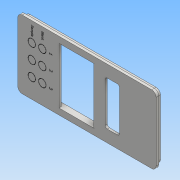
# Autodesk Inventor part: Box2_top
Saved by Autodesk Inventor 2016 (Build 200138000, 138)
## iProperties
Created: 2015-09-13
Part Number: Box2_top
Material: PPS Plastic
Document SubType Name: Modeling
Designer: Openlab
Density: 1.637 g/cm^3
Appearance: White
Mass: 58.6735 g
Surface Area: 261.578 cm^2
Volume: 35.8421 cm^3
Author: Openlab
Autodesk Inventor part; units mm, degrees
(part 1 of 2)
ref_plane "YZ Plane" through (0, 0, 0) normal (1, 0, 0) x (0, 1, 0)
ref_plane "XZ Plane" through (0, 0, 0) normal (0, 1, 0) x (-1, 0, 0)
ref_plane "XY Plane" through (0, 0, 0) normal (0, 0, 1) x (1, 0, 0)
sketch "Sketch1" plane through (0, 0, 0) normal (0, 1, 0) x (-1, 0, 0)
  line L0 (-70, 35) -> (70, 35)
  line L1 (75, 30) -> (75, -30)
  line L2 (70, -35) -> (-70, -35)
  line L3 (-75, -30) -> (-75, 30)
  line L4 (-75, 35) -> (75, -35) construction
  line L5 (75, 35) -> (-75, -35) construction
  arc A0 (75, 30) -> (70, 35) centre (70, 30) ccw
  arc A1 (70, -35) -> (75, -30) centre (70, -30) ccw
  arc A2 (-70, 35) -> (-75, 30) centre (-70, 30) ccw
  arc A3 (-75, -30) -> (-70, -35) centre (-70, -30) ccw
  line L6 (-72, 37) -> (72, 37)
  line L7 (77, 32) -> (77, -32)
  line L8 (72, -37) -> (-72, -37)
  line L9 (-77, -32) -> (-77, 32)
  line L10 (-77, 37) -> (77, -37) construction
  line L11 (77, 37) -> (-77, -37) construction
  arc A4 (77, 32) -> (72, 37) centre (72, 32) ccw
  arc A5 (72, -37) -> (77, -32) centre (72, -32) ccw
  arc A6 (-77, -32) -> (-72, -37) centre (-72, -32) ccw
  arc A7 (-72, 37) -> (-77, 32) centre (-72, 32) ccw
  line L12 (74, 39) -> (-74, 39)
  line L13 (-79, 34) -> (-79, -34)
  line L14 (-74, -39) -> (74, -39)
  line L15 (79, -34) -> (79, 34)
  line L16 (79, 39) -> (-79, -39) construction
  line L17 (-79, 39) -> (79, -39) construction
  arc A8 (79, 34) -> (74, 39) centre (74, 34) ccw
  arc A9 (-74, 39) -> (-79, 34) centre (-74, 34) ccw
  arc A10 (-79, -34) -> (-74, -39) centre (-74, -34) ccw
  arc A11 (74, -39) -> (79, -34) centre (74, -34) ccw
  line L18 (-22.75, 23.25) -> (-35.25, 23.25) construction
  line L19 (-35.25, 23.25) -> (-35.25, 19) construction
  line L20 (-35.25, 10.75) -> (-22.75, 10.75) construction
  line L21 (-22.75, 10.75) -> (-22.75, 15) construction
  line L22 (56.9183, 17) -> (21.35, 17) construction
  line L23 (40.8, -24) -> (40.8, -20.1) construction
  line L24 (-55.8, 24) -> (-55.8, 12) construction
  line L25 (-20.25, 15.5) -> (-22.25, 15.5) construction
  line L26 (-22.25, 18.5) -> (-20.25, 18.5) construction
  line L27 (-35.75, 15.5) -> (-37.75, 15.5) construction
  line L28 (-37.75, 18.5) -> (-35.75, 18.5) construction
  line L29 (-40.55, 18.5) -> (-53.5, 18.5) construction
  line L30 (-40.55, 15.5) -> (-53.5, 15.5) construction
  line L31 (-60, 8.5) -> (45, 8.5) construction
  line L32 (38.5, 20.5) -> (37, 20.5) construction
  line L33 (37, 13.5) -> (38.5, 13.5) construction
  line L34 (-60, 5) -> (-60, -25) construction
  line L35 (21.35, -8.5) -> (45, -8.5) construction
  line L36 (-29, 20.0147) -> (-29, -25.5) construction
  line L37 (31.2062, 0) -> (-4.2501, 0) construction
  line L38 (-35.25, 6.25) -> (-35.25, 2) construction
  line L39 (-22.75, 6.25) -> (-35.25, 6.25) construction
  line L40 (-22.75, -6.25) -> (-22.75, -2) construction
  line L41 (-35.25, -6.25) -> (-22.75, -6.25) construction
  line L42 (-22.25, 1.5) -> (-20.25, 1.5) construction
  line L43 (-20.25, -1.5) -> (-22.25, -1.5) construction
  line L44 (38.5, 3.5) -> (37, 3.5) construction
  line L45 (37, -3.5) -> (38.5, -3.5) construction
  line L46 (-22.75, -10.75) -> (-35.25, -10.75) construction
  line L47 (-22.75, -23.25) -> (-22.75, -19) construction
  line L48 (-35.25, -23.25) -> (-22.75, -23.25) construction
  line L49 (56.3008, -17) -> (21.35, -17) construction
  line L50 (38.5, -13.5) -> (37, -13.5) construction
  line L51 (37, -20.5) -> (38.5, -20.5) construction
  line L52 (-20.25, -18.5) -> (-22.25, -18.5) construction
  line L53 (44.5, 5.5) -> (43.5, 5.5) construction
  line L54 (41.3, 11.5) -> (43.5, 11.5) construction
  line L55 (-37.75, -15.5) -> (-35.75, -15.5) construction
  line L56 (-35.75, -18.5) -> (-37.75, -18.5) construction
  line L57 (-40.55, -18.5) -> (-53.5, -18.5) construction
  line L58 (-37.75, 1.5) -> (-35.75, 1.5) construction
  line L59 (-35.75, -1.5) -> (-37.75, -1.5) construction
  line L60 (-40.55, -1.5) -> (-53.5, -1.5) construction
  line L61 (-58.5, 5.5) -> (-59.5, 5.5) construction
  line L62 (-59.5, 11.5) -> (-58.5, 11.5) construction
  line L63 (38.5, 5.5) -> (37, 5.5) construction
  line L64 (37, 5.5) -> (37, 11.5) construction
  line L65 (37, 11.5) -> (38.5, 11.5) construction
  line L66 (-53.5, 5.5) -> (-52.5, 5.5) construction
  line L67 (-52.5, 5.5) -> (-52.5, 11.5) construction
  line L68 (-52.5, 11.5) -> (-53.5, 11.5) construction
  line L69 (-54, 24) -> (-54, 19) construction
  line L70 (-54, 5) -> (-54, 2) construction
  arc A12 (-12.95, 13.5) -> (-12.95, 3.5) centre (-12.95, 8.5) ccw construction
  arc A13 (31, 3.5) -> (31, 13.5) centre (31, 8.5) ccw construction
  arc A14 (-12.95, -3.5) -> (-12.95, -13.5) centre (-12.95, -8.5) ccw construction
  arc A15 (31, -13.5) -> (31, -3.5) centre (31, -8.5) ccw construction
  line L71 (-12.95, 13.5) -> (31, 13.5) construction
  line L72 (-12.95, 3.5) -> (31, 3.5) construction
  line L73 (-12.95, -3.5) -> (31, -3.5) construction
  line L74 (-12.95, -13.5) -> (31, -13.5) construction
  arc A16 (-45.05, -13.5) -> (-45.05, -3.5) centre (-45.05, -8.5) ccw construction
  line L75 (43.5, -24) -> (43.5, -19.6) construction
  line L76 (-58.5, 24) -> (-58.5, 11.5) construction
  arc A17 (-46, -3.5) -> (-46, -13.5) centre (-46, -8.5) ccw construction
  arc A18 (-46, 13.5) -> (-46, 3.5) centre (-46, 8.5) ccw construction
  line L77 (-45.05, -13.5) -> (-46, -13.5) construction
  line L78 (-46, -3.5) -> (-45.05, -3.5) construction
  line L79 (-46, 3.5) -> (-45.05, 3.5) construction
  line L80 (-45.05, 13.5) -> (-46, 13.5) construction
  arc A19 (-45.05, 3.5) -> (-45.05, 13.5) centre (-45.05, 8.5) ccw construction
  line L81 (29.8763, -15.5) -> (-17.45, -15.5) construction
  line L82 (29.8763, -18.5) -> (-17.45, -18.5) construction
  line L83 (29.8763, -1.5) -> (-17.45, -1.5) construction
  line L84 (29.8763, 1.5) -> (-17.45, 1.5) construction
  line L85 (29.8763, 15.5) -> (-17.45, 15.5) construction
  line L86 (29.8763, 18.5) -> (-17.45, 18.5) construction
  arc A20 (32, -14.4) -> (29.8763, -15.5) centre (32, -17) ccw construction
  arc A21 (29.8763, -18.5) -> (32, -19.6) centre (32, -17) ccw construction
  arc A22 (32, 2.6) -> (29.8763, 1.5) centre (32, 0) ccw construction
  arc A23 (29.8763, -1.5) -> (32, -2.6) centre (32, 0) ccw construction
  arc A24 (32, 19.6) -> (29.8763, 18.5) centre (32, 17) ccw construction
  arc A25 (29.8763, 15.5) -> (32, 14.4) centre (32, 17) ccw construction
  arc A26 (34.4725, -25.0625) -> (31, -22) centre (31, -25.5) ccw construction
  arc A27 (-12.95, -22) -> (-16.4225, -25.0625) centre (-12.95, -25.5) ccw construction
  arc A28 (35.7697, -24) -> (31, -20.5) centre (31, -25.5) ccw construction
  line L87 (31, -20.5) -> (-12.95, -20.5) construction
  line L88 (34.9686, -25.5) -> (44.5, -25.5) construction
  line L89 (31, -22) -> (-12.95, -22) construction
  arc A29 (-12.95, -20.5) -> (-17.7197, -24) centre (-12.95, -25.5) ccw construction
  arc A30 (-17.6941, 23.9209) -> (-12.95, 20.5) centre (-12.95, 25.5) ccw construction
  arc A31 (-16.4225, 25.0625) -> (-12.95, 22) centre (-12.95, 25.5) ccw construction
  line L90 (31, 22) -> (-12.95, 22) construction
  line L91 (31, 20.5) -> (-12.95, 20.5) construction
  line L92 (35.7697, 24) -> (40.8, 24) construction
  line L93 (44.5, 25.5) -> (34.9686, 25.5) construction
  arc A32 (31, 22) -> (34.4725, 25.0625) centre (31, 25.5) ccw construction
  arc A33 (31, 20.5) -> (35.7697, 24) centre (31, 25.5) ccw construction
  arc A34 (-41.5775, -25.0625) -> (-45.05, -22) centre (-45.05, -25.5) ccw construction
  arc A35 (-46, -22) -> (-49.4725, -25.0625) centre (-46, -25.5) ccw construction
  line L94 (-45.05, -20.5) -> (-46, -20.5) construction
  line L95 (-45.05, -22) -> (-46, -22) construction
  arc A36 (-46, -20.5) -> (-50.7697, -24) centre (-46, -25.5) ccw construction
  arc A37 (-40.2803, -24) -> (-45.05, -20.5) centre (-45.05, -25.5) ccw construction
  line L96 (-17.7197, -24) -> (-40.2803, -24) construction
  line L97 (-50.7697, -24) -> (-58.5, -24) construction
  line L98 (-59.5, -25.5) -> (-49.9686, -25.5) construction
  line L99 (-17.2197, -25.5) -> (-16.9186, -25.5) construction
  line L100 (-45.05, 20.5) -> (-46, 20.5) construction
  line L101 (-45.05, 22) -> (-46, 22) construction
  arc A38 (-49.4725, 25.0625) -> (-46, 22) centre (-46, 25.5) ccw construction
  arc A39 (-45.05, 22) -> (-41.5775, 25.0625) centre (-45.05, 25.5) ccw construction
  arc A40 (-50.7697, 24) -> (-46, 20.5) centre (-46, 25.5) ccw construction
  arc A41 (-45.05, 20.5) -> (-40.336, 23.8333) centre (-45.05, 25.5) ccw construction
  line L102 (-16.9186, 25.5) -> (-17.2197, 25.5) construction
  line L103 (-49.9686, 25.5) -> (-59.5, 25.5) construction
  line L104 (-58.5, 24) -> (-50.7697, 24) construction
  line L105 (-40.3074, 24) -> (-17.7197, 24) construction
  line L106 (-17.7197, -24) -> (-17.7197, -25) construction
  line L107 (-40.2803, -24) -> (-40.2803, -25) construction
  line L108 (-40.3074, 24) -> (-40.3074, 25) construction
  line L109 (-17.7197, 24.0788) -> (-17.7197, 25) construction
  line L110 (43.5, 11.5) -> (44.5, 11.5) construction
  line L111 (43.5, 5.5) -> (41.3, 5.5) construction
  line L112 (-56.3, 11.5) -> (-58.5, 11.5) construction
  line L113 (-56.3, 5.5) -> (-58.5, 5.5) construction
  line L114 (-17.95, -21) -> (-19.75, -21) construction
  line L115 (-19.75, -13) -> (-17.95, -13) construction
  line L116 (-17.95, -4) -> (-19.75, -4) construction
  line L117 (-19.75, 4) -> (-17.95, 4) construction
  line L118 (-17.95, 13) -> (-19.75, 13) construction
  line L119 (-19.75, 21) -> (-17.95, 21) construction
  line L120 (-38.25, -21) -> (-40.05, -21) construction
  line L121 (-40.05, -13) -> (-38.25, -13) construction
  line L122 (-38.25, -4) -> (-40.05, -4) construction
  line L123 (-40.05, 4) -> (-38.25, 4) construction
  line L124 (-38.25, 13) -> (-40.05, 13) construction
  line L125 (-40.05, 21) -> (-38.25, 21) construction
  line L126 (-17.95, -13) -> (-17.95, -15) construction
  line L127 (-17.95, -19) -> (-17.95, -21) construction
  line L128 (-19.75, -21) -> (-19.75, -19) construction
  line L129 (-17.95, 4) -> (-17.95, 2) construction
  line L130 (-17.95, -2) -> (-17.95, -4) construction
  line L131 (-19.75, -4) -> (-19.75, -2) construction
  line L132 (-19.75, 2) -> (-19.75, 4) construction
  line L133 (-17.95, 21) -> (-17.95, 19) construction
  line L134 (-17.95, 15) -> (-17.95, 13) construction
  line L135 (-19.75, 13) -> (-19.75, 15) construction
  line L136 (-19.75, 19) -> (-19.75, 21) construction
  line L137 (-38.25, -13) -> (-38.25, -15) construction
  line L138 (-38.25, -19) -> (-38.25, -21) construction
  line L139 (-40.05, -21) -> (-40.05, -19) construction
  line L140 (-40.05, -15) -> (-40.05, -13) construction
  line L141 (-38.25, 4) -> (-38.25, 2) construction
  line L142 (-38.25, -2) -> (-38.25, -4) construction
  line L143 (-40.05, -4) -> (-40.05, -2) construction
  line L144 (-40.05, 2) -> (-40.05, 4) construction
  line L145 (-38.25, 21) -> (-38.25, 19) construction
  line L146 (-38.25, 15) -> (-38.25, 13) construction
  line L147 (-40.05, 13) -> (-40.05, 15) construction
  line L148 (-40.05, 19) -> (-40.05, 21) construction
  line L149 (38.5, -11.5) -> (37, -11.5) construction
  line L150 (37, -11.5) -> (37, -5.5) construction
  line L151 (37, -5.5) -> (38.5, -5.5) construction
  line L152 (39, -21) -> (39, -24) construction
  arc A42 (-19.75, -19) -> (-20.25, -18.5) centre (-20.25, -19) ccw construction
  arc A43 (-17.45, -18.5) -> (-17.95, -19) centre (-17.45, -19) ccw construction
  arc A44 (-19.75, -2) -> (-20.25, -1.5) centre (-20.25, -2) ccw construction
  arc A45 (-17.45, -1.5) -> (-17.95, -2) centre (-17.45, -2) ccw construction
  arc A46 (-17.95, 2) -> (-17.45, 1.5) centre (-17.45, 2) ccw construction
  arc A47 (-20.25, 1.5) -> (-19.75, 2) centre (-20.25, 2) ccw construction
  arc A48 (-19.75, 15) -> (-20.25, 15.5) centre (-20.25, 15) ccw construction
  arc A49 (-17.45, 15.5) -> (-17.95, 15) centre (-17.45, 15) ccw construction
  arc A50 (-17.95, 19) -> (-17.45, 18.5) centre (-17.45, 19) ccw construction
  arc A51 (-20.25, 18.5) -> (-19.75, 19) centre (-20.25, 19) ccw construction
  arc A52 (-38.25, 19) -> (-37.75, 18.5) centre (-37.75, 19) ccw construction
  arc A53 (-40.55, 18.5) -> (-40.05, 19) centre (-40.55, 19) ccw construction
  arc A54 (-40.05, 15) -> (-40.55, 15.5) centre (-40.55, 15) ccw construction
  arc A55 (-37.75, 15.5) -> (-38.25, 15) centre (-37.75, 15) ccw construction
  arc A56 (-38.25, 2) -> (-37.75, 1.5) centre (-37.75, 2) ccw construction
  arc A57 (-40.55, 1.5) -> (-40.05, 2) centre (-40.55, 2) ccw construction
  arc A58 (-40.05, -2) -> (-40.55, -1.5) centre (-40.55, -2) ccw construction
  arc A59 (-37.75, -1.5) -> (-38.25, -2) centre (-37.75, -2) ccw construction
  arc A60 (-38.25, -15) -> (-37.75, -15.5) centre (-37.75, -15) ccw construction
  arc A61 (-40.55, -15.5) -> (-40.05, -15) centre (-40.55, -15) ccw construction
  arc A62 (-37.75, -18.5) -> (-38.25, -19) centre (-37.75, -19) ccw construction
  arc A63 (-40.05, -19) -> (-40.55, -18.5) centre (-40.55, -19) ccw construction
  line L153 (36.5, -19.6) -> (32, -19.6) construction
  line L154 (37, -13.5) -> (37, -13.9) construction
  line L155 (32, -14.4) -> (36.5, -14.4) construction
  line L156 (36.5, -2.6) -> (32, -2.6) construction
  line L157 (37, 3.5) -> (37, 3.1) construction
  line L158 (37, -3.1) -> (37, -3.5) construction
  line L159 (32, 2.6) -> (36.5, 2.6) construction
  line L160 (36.5, 14.4) -> (32, 14.4) construction
  line L161 (37, 20.5) -> (37, 20.1) construction
  line L162 (37, 13.9) -> (37, 13.5) construction
  line L163 (32, 19.6) -> (36.5, 19.6) construction
  arc A64 (36.5, -14.4) -> (37, -13.9) centre (36.5, -13.9) ccw construction
  arc A65 (39, -12) -> (38.5, -11.5) centre (38.5, -12) ccw construction
  arc A66 (38.5, -5.5) -> (39, -5) centre (38.5, -5) ccw construction
  arc A67 (39, 5) -> (38.5, 5.5) centre (38.5, 5) ccw construction
  arc A68 (38.5, 11.5) -> (39, 12) centre (38.5, 12) ccw construction
  arc A69 (37, -3.1) -> (36.5, -2.6) centre (36.5, -3.1) ccw construction
  arc A70 (36.5, 2.6) -> (37, 3.1) centre (36.5, 3.1) ccw construction
  arc A71 (37, 13.9) -> (36.5, 14.4) centre (36.5, 13.9) ccw construction
  arc A72 (36.5, 19.6) -> (37, 20.1) centre (36.5, 20.1) ccw construction
  line L164 (43.5, -2.6) -> (43.5, 2.6) construction
  line L165 (43.5, -2.6) -> (41.3, -2.6) construction
  line L166 (37, -20.5) -> (37, -20.1) construction
  arc A73 (37, -20.1) -> (36.5, -19.6) centre (36.5, -20.1) ccw construction
  line L167 (39, -13) -> (39, -12) construction
  line L168 (39, 4) -> (39, 5) construction
  line L169 (39, 21) -> (39, 24) construction
  line L170 (43.5, -19.6) -> (43.5, -14.4) construction
  line L171 (43.5, -19.6) -> (41.3, -19.6) construction
  line L172 (43.5, -24) -> (40.8, -24) construction
  line L173 (40.8, -24) -> (39, -24) construction
  line L174 (39, -24) -> (35.7697, -24) construction
  line L175 (41.3, -14.4) -> (43.5, -14.4) construction
  line L176 (43.5, -14.4) -> (43.5, -2.6) construction
  line L177 (40.8, -13.9) -> (40.8, -3.1) construction
  line L178 (39, -4) -> (39, -5) construction
  line L179 (43.5, 2.6) -> (43.5, 5.5) construction
  line L180 (41.3, 2.6) -> (43.5, 2.6) construction
  line L181 (40.8, 3.1) -> (40.8, 5) construction
  line L182 (43.5, 14.4) -> (43.5, 19.6) construction
  line L183 (43.5, 14.4) -> (41.3, 14.4) construction
  line L184 (45, -25) -> (45, 5) construction
  line L185 (43.5, 19.6) -> (43.5, 24) construction
  line L186 (40.8, 20.1) -> (40.8, 24) construction
  line L187 (41.3, 19.6) -> (43.5, 19.6) construction
  line L188 (43.5, 11.5) -> (43.5, 14.4) construction
  line L189 (40.8, 24) -> (43.5, 24) construction
  line L190 (40.8, 12) -> (40.8, 13.9) construction
  line L191 (39, 13) -> (39, 12) construction
  arc A74 (38.5, -13.5) -> (39, -13) centre (38.5, -13) ccw construction
  arc A75 (39, -4) -> (38.5, -3.5) centre (38.5, -4) ccw construction
  arc A76 (38.5, 3.5) -> (39, 4) centre (38.5, 4) ccw construction
  arc A77 (39, 13) -> (38.5, 13.5) centre (38.5, 13) ccw construction
  arc A78 (38.5, 20.5) -> (39, 21) centre (38.5, 21) ccw construction
  arc A79 (41.3, -19.6) -> (40.8, -20.1) centre (41.3, -20.1) ccw construction
  arc A80 (40.8, -13.9) -> (41.3, -14.4) centre (41.3, -13.9) ccw construction
  arc A81 (41.3, -2.6) -> (40.8, -3.1) centre (41.3, -3.1) ccw construction
  arc A82 (40.8, 3.1) -> (41.3, 2.6) centre (41.3, 3.1) ccw construction
  arc A83 (41.3, 14.4) -> (40.8, 13.9) centre (41.3, 13.9) ccw construction
  arc A84 (40.8, 20.1) -> (41.3, 19.6) centre (41.3, 20.1) ccw construction
  line L192 (40.8, 5.5) -> (40.8, 11.5) construction
  line L193 (-54, 15) -> (-54, 12) construction
  line L194 (-53.5, 1.5) -> (-40.55, 1.5) construction
  line L195 (-54, -2) -> (-54, -15) construction
  line L196 (-54, -19) -> (-54, -24) construction
  line L197 (-53.5, -15.5) -> (-40.55, -15.5) construction
  line L198 (-58.5, 5.5) -> (-58.5, -24) construction
  arc A85 (-54, 19) -> (-53.5, 18.5) centre (-53.5, 19) ccw construction
  arc A86 (-53.5, 15.5) -> (-54, 15) centre (-53.5, 15) ccw construction
  arc A87 (-54, 12) -> (-53.5, 11.5) centre (-53.5, 12) ccw construction
  arc A88 (-53.5, 5.5) -> (-54, 5) centre (-53.5, 5) ccw construction
  arc A89 (-54, 2) -> (-53.5, 1.5) centre (-53.5, 2) ccw construction
  arc A90 (-53.5, -1.5) -> (-54, -2) centre (-53.5, -2) ccw construction
  arc A91 (-54, -15) -> (-53.5, -15.5) centre (-53.5, -15) ccw construction
  arc A92 (-53.5, -18.5) -> (-54, -19) centre (-53.5, -19) ccw construction
  arc A93 (39, -21) -> (38.5, -20.5) centre (38.5, -21) ccw construction
  arc A94 (41.3, 5.5) -> (40.8, 5) centre (41.3, 5) ccw construction
  arc A95 (40.8, 12) -> (41.3, 11.5) centre (41.3, 12) ccw construction
  line L199 (40.8, 5.5) -> (41.3, 5.5) construction
  line L200 (40.8, 11.5) -> (41.3, 11.5) construction
  arc A96 (45, 5) -> (44.5, 5.5) centre (44.5, 5) ccw construction
  line L201 (45, 25) -> (45, 12) construction
  arc A97 (44.5, 11.5) -> (45, 12) centre (44.5, 12) ccw construction
  line L202 (45, 5) -> (45, 12) construction
  arc A98 (-59.5, 5.5) -> (-60, 5) centre (-59.5, 5) ccw construction
  line L203 (-60, 12) -> (-60, 25) construction
  arc A99 (-60, 12) -> (-59.5, 11.5) centre (-59.5, 12) ccw construction
  line L204 (-60, 5) -> (-60, 12) construction
  line L205 (-55.8, -24) -> (-55.8, 5) construction
  arc A100 (-56.3, 11.5) -> (-55.8, 12) centre (-56.3, 12) ccw construction
  arc A101 (-55.8, 5) -> (-56.3, 5.5) centre (-56.3, 5) ccw construction
  line L206 (-55.8, 5.5) -> (-55.8, 11.5) construction
  line L207 (-56.3, 11.5) -> (-55.8, 11.5) construction
  line L208 (-56.3, 5.5) -> (-55.8, 5.5) construction
  arc A102 (44.5, -25.5) -> (45, -25) centre (44.5, -25) ccw construction
  arc A103 (34.4725, -25.0625) -> (34.9686, -25.5) centre (34.9686, -25) ccw construction
  arc A104 (-16.9186, -25.5) -> (-16.4225, -25.0625) centre (-16.9186, -25) ccw construction
  arc A105 (-41.5775, -25.0625) -> (-41.0814, -25.5) centre (-41.0814, -25) ccw construction
  arc A106 (-49.9686, -25.5) -> (-49.4725, -25.0625) centre (-49.9686, -25) ccw construction
  arc A107 (-60, -25) -> (-59.5, -25.5) centre (-59.5, -25) ccw construction
  arc A108 (-59.5, 25.5) -> (-60, 25) centre (-59.5, 25) ccw construction
  arc A109 (-49.4725, 25.0625) -> (-49.9686, 25.5) centre (-49.9686, 25) ccw construction
  arc A110 (-41.0814, 25.5) -> (-41.5775, 25.0625) centre (-41.0814, 25) ccw construction
  arc A111 (-16.4225, 25.0625) -> (-16.9186, 25.5) centre (-16.9186, 25) ccw construction
  arc A112 (34.9686, 25.5) -> (34.4725, 25.0625) centre (34.9686, 25) ccw construction
  arc A113 (45, 25) -> (44.5, 25.5) centre (44.5, 25) ccw construction
  line L209 (-22.75, -19) -> (-22.75, -15) construction
  line L210 (-22.75, -15) -> (-22.75, -10.75) construction
  line L211 (-35.25, -15) -> (-35.25, -19) construction
  line L212 (-35.25, -19) -> (-35.25, -23.25) construction
  arc A114 (-22.25, -18.5) -> (-22.75, -19) centre (-22.25, -19) ccw construction
  arc A115 (-22.75, -15) -> (-22.25, -15.5) centre (-22.25, -15) ccw construction
  arc A116 (-35.25, -19) -> (-35.75, -18.5) centre (-35.75, -19) ccw construction
  arc A117 (-17.95, -15) -> (-17.45, -15.5) centre (-17.45, -15) ccw construction
  line L213 (-19.75, -13) -> (-19.75, -15) construction
  line L214 (-20.25, -15.5) -> (-22.25, -15.5) construction
  arc A118 (-20.25, -15.5) -> (-19.75, -15) centre (-20.25, -15) ccw construction
  line L215 (-35.25, -10.75) -> (-35.25, -15) construction
  arc A119 (-35.75, -15.5) -> (-35.25, -15) centre (-35.75, -15) ccw construction
  line L216 (-22.75, -2) -> (-22.75, 2) construction
  line L217 (-22.75, 2) -> (-22.75, 6.25) construction
  line L218 (-35.25, -2) -> (-35.25, -6.25) construction
  line L219 (-35.25, 2) -> (-35.25, -2) construction
  line L220 (-22.75, 15) -> (-22.75, 19) construction
  line L221 (-22.75, 19) -> (-22.75, 23.25) construction
  line L222 (-35.25, 19) -> (-35.25, 15) construction
  line L223 (-35.25, 15) -> (-35.25, 10.75) construction
  arc A120 (-22.25, -1.5) -> (-22.75, -2) centre (-22.25, -2) ccw construction
  arc A121 (-22.75, 2) -> (-22.25, 1.5) centre (-22.25, 2) ccw construction
  arc A122 (-35.25, -2) -> (-35.75, -1.5) centre (-35.75, -2) ccw construction
  arc A123 (-35.75, 1.5) -> (-35.25, 2) centre (-35.75, 2) ccw construction
  arc A124 (-22.25, 15.5) -> (-22.75, 15) centre (-22.25, 15) ccw construction
  arc A125 (-22.75, 19) -> (-22.25, 18.5) centre (-22.25, 19) ccw construction
  arc A126 (-35.75, 18.5) -> (-35.25, 19) centre (-35.75, 19) ccw construction
  arc A127 (-35.25, 15) -> (-35.75, 15.5) centre (-35.75, 15) ccw construction
  arc A128 (-17.7197, -25) -> (-17.2197, -25.5) centre (-17.2197, -25) ccw construction
  line L224 (-41.0814, -25.5) -> (-40.7803, -25.5) construction
  line L225 (-40.7803, -25.5) -> (-17.2197, -25.5) construction
  arc A129 (-40.7803, -25.5) -> (-40.2803, -25) centre (-40.7803, -25) ccw construction
  arc A130 (-17.2197, 25.5) -> (-17.7197, 25) centre (-17.2197, 25) ccw construction
  line L226 (-41.0814, 25.5) -> (-40.8074, 25.5) construction
  line L227 (-40.8074, 25.5) -> (-17.2197, 25.5) construction
  arc A131 (-40.3074, 25) -> (-40.8074, 25.5) centre (-40.8074, 25) ccw construction
  arc A132 (-17.7197, 24.0788) -> (-17.6941, 23.9209) centre (-17.2197, 24.0788) ccw construction
  arc A133 (-40.336, 23.8333) -> (-40.3074, 24) centre (-40.8074, 24) ccw construction
  line L228 (-23.25, 25.25) -> (-34.75, 25.25)
  line L229 (-37.25, 22.75) -> (-37.25, -22.75)
  line L230 (-34.75, -25.25) -> (-23.25, -25.25)
  line L231 (-20.75, -22.75) -> (-20.75, 22.75)
  line L232 (-20.75, 25.25) -> (-37.25, -25.25) construction
  line L233 (-37.25, 25.25) -> (-20.75, -25.25) construction
  arc A134 (-23.25, -25.25) -> (-20.75, -22.75) centre (-23.25, -22.75) ccw
  arc A135 (-37.25, -22.75) -> (-34.75, -25.25) centre (-34.75, -22.75) ccw
  arc A136 (-20.75, 22.75) -> (-23.25, 25.25) centre (-23.25, 22.75) ccw
  arc A137 (-34.75, 25.25) -> (-37.25, 22.75) centre (-34.75, 22.75) ccw
  line L234 (67, 32) -> (-67, 32)
  line L235 (-72, 27) -> (-72, -27)
  line L236 (-67, -32) -> (67, -32)
  line L237 (72, -27) -> (72, 27)
  line L238 (72, 32) -> (-72, -32) construction
  line L239 (-72, 32) -> (72, -32) construction
  arc A138 (67, -32) -> (72, -27) centre (67, -27) ccw
  arc A139 (-72, -27) -> (-67, -32) centre (-67, -27) ccw
  arc A140 (-67, 32) -> (-72, 27) centre (-67, 27) ccw
  arc A141 (72, 27) -> (67, 32) centre (67, 27) ccw
  line L240 (31.8988, -34.35) -> (-8.0012, -34.35)
  line L241 (-8.0012, -34.35) -> (-8.0012, 34.35)
  line L242 (-8.0012, 34.35) -> (31.8988, 34.35)
  line L243 (31.8988, 34.35) -> (31.8988, -34.35)
  line L244 (31.8988, -34.35) -> (-8.0012, 34.35) construction
  line L245 (-8.0012, -34.35) -> (31.8988, 34.35) construction
  point P0 (0, 0)
  point P1 (0, 0)
  point P2 (0, 0)
  point P3 (-29, -17)
  point P4 (-29, 0)
  point P5 (-29, 17)
  point P6 (43.5, -8.5)
  point P7 (11.9488, 0)
  point P8 (11.9488, 0)
  dimension "d0" = 150
  dimension "d1" = 70
  dimension "d2" = 5
  dimension "d3" = 2
  dimension "d4" = 2
  dimension "d5" = 5
  dimension "d6" = 4
  dimension "d7" = 4
  dimension "d8" = 5
  dimension "d13" = 7
  dimension "d14" = 17
  dimension "d15" = 17
  dimension "d16" = 17
  dimension "d17" = 6
  dimension "d18" = 6
  dimension "d19" = 5
  dimension "d20" = 1.5
  dimension "d21" = 1.5
  dimension "d22" = 1.5
  dimension "d23" = 17
  dimension "d24" = 17
  dimension "d25" = 2.7
  dimension "d26" = 2.7
  dimension "d27" = 6
  dimension "d28" = 25
  dimension "d29" = 5
  dimension "d30" = 1.8
  dimension "d31" = 8
  dimension "d32" = 5
  dimension "d33" = 5
  dimension "d34" = 12.5
  dimension "d35" = 51
  dimension "d36" = 8
  dimension "d37" = 7
  dimension "d38" = 7
  dimension "d39" = 2
  dimension "d40" = 1.8
  dimension "d41" = 8
  dimension "d42" = 1.8
  dimension "d43" = 2.7
  dimension "d44" = 1.5
  dimension "d45" = 3
  dimension "d46" = 3
  dimension "d47" = 3
  dimension "d48" = 0.5
  dimension "d49" = 68
  dimension "d50" = 5.2
  dimension "d51" = 7
  dimension "d52" = 5.2
  dimension "d53" = 5.2
  dimension "d54" = 1.5
  dimension "d55" = 1.5
  dimension "d56" = 0.5
  dimension "d57" = 0.5
  dimension "d58" = 0.5
  dimension "d59" = 6
  dimension "d60" = 0.5
  dimension "d61" = 12.5
  dimension "d62" = 3
  dimension "d63" = 3
  dimension "d64" = 12.5
  dimension "d65" = 12.5
  dimension "d66" = 0.5
  dimension "d67" = 0.5
  constraints: 494 end point, 287 point on circle, 265 tangent, 169 perpendicular, 142 centre point, 124 equal radius, 111 collinear, 81 parallel, 75 point on line, 35 horizontal, 15 midpoint, 14 vertical alignment, 10 coincident, 9 vertical, 7 horizontal alignment, 38 other
  measures "d0" distance of L4.end L5.end
  measures "d1" distance of L5.start L4.end
  measures "d2" radius of A0
  measures "d3" distance between parallel lines of L8 L2
  measures "d4" distance between parallel lines of L7 L1
  measures "d5" radius of A4
  measures "d6" distance between parallel lines of L15 L1
  measures "d7" distance between parallel lines of L14 L2
  measures "d8" radius of A8
  measures "d13" distance of L32.end L33.start
  measures "d14" distance between parallel lines of L37 L22
  measures "d15" distance between parallel lines of L49 L37
  measures "d16" distance between parallel lines of L31 L35
  measures "d17" distance of L63.end L64.end
  measures "d18" distance of L66.end L67.end
  measures "d19" radius of A28
  measures "d20" radial gap between concentric circles of A26 A28
  measures "d21" distance between parallel lines of L93 L92
  measures "d22" distance between parallel lines of L97 L98
  measures "d23" distance between parallel lines of L35 L98
  measures "d24" distance between parallel lines of L103 L31
  measures "d25" distance between parallel lines of L76 L24
  measures "d26" distance between parallel lines of L23 L75
  measures "d27" distance between parallel lines of L111 L54
  measures "d28" distance between parallel lines of L69 L36
  measures "d29" radius of A14
  measures "d30" distance of L114.start L114.end
  measures "d31" distance between parallel lines of L115 L114
  measures "d32" distance from line of A27.centre L127
  measures "d33" distance from line of A37.centre L139
  measures "d34" distance between parallel lines of L18 L20
  measures "d35" distance between parallel lines of L93 L88
  measures "d36" distance from line of A26.centre L152
  measures "d37" distance between parallel lines of L44 L45
  measures "d38" distance between parallel lines of L50 L51
  measures "d39" distance between parallel lines of L64 L168
  measures "d40" distance between parallel lines of L152 L23
  measures "d41" distance from line of L196 A36.centre
  measures "d42" distance between parallel lines of L24 L196
  measures "d43" distance between parallel lines of L198 L24
  measures "d44" distance between parallel lines of L34 L198
  measures "d45" distance between parallel lines of L197 L57
  measures "d46" distance between parallel lines of L60 L194
  measures "d47" distance between parallel lines of L29 L30
  measures "d48" radius of A44
  measures "d49" distance between parallel lines of L169 L36
  measures "d50" distance between parallel lines of L175 L171
  measures "d51" distance from line of A22.centre L178
  measures "d52" distance between parallel lines of L180 L165
  measures "d53" distance between parallel lines of L187 L183
  measures "d54" distance between parallel lines of L70 L67
  measures "d55" distance between parallel lines of L75 L184
  measures "d56" radius of A94
  measures "d57" radius of A96
  measures "d58" radius of A97
  measures "d59" distance between parallel lines of L62 L61
  measures "d60" radius of A102
  measures "d61" distance between parallel lines of L46 L48
  measures "d62" distance between parallel lines of L47 L128
  measures "d63" distance between parallel lines of L138 L212
  measures "d64" distance between parallel lines of L39 L41
  measures "d65" distance between parallel lines of L223 L21
  measures "d66" radius of A128
  measures "d67" radius of A129
extrude "Extrusion1" add sketch "Sketch1" along normal blind 7 contours L0 A0 L1 A1 L2 A3 L3 A2 | L6 A4 L7 A5 L8 A6 L9 A7 | L234 L241 L242 L243 | L243 L240 L241 L236
extrude "Extrusion2" add sketch "Sketch1" along normal blind 3 contours A8 L15 A11 L14 A10 L13 A9 L12
extrude "Extrusion3" add sketch "Sketch1" along normal blind 2.5 contours A141 L237 A138 L236 L243 L234 | L241 L236 A139 L235 A140 L234
sketch "Sketch2" plane through (0, 0, 0) normal (0, -1, 0) x (1, 0, 0)
  circle A0 centre (-51, 17) radius 4
  circle A1 centre (-51, 0) radius 4
  circle A2 centre (-51, -17) radius 4
  circle A3 centre (-63, 17) radius 4
  circle A4 centre (-63, 0) radius 4
  circle A5 centre (-63, -17) radius 4
  line L0 (-32.0282, 0) -> (-24.8059, 0) construction
  line L1 (-74, 39) -> (74, 39) construction
  line L2 (74, -39) -> (-74, -39) construction
  line L3 (-79, -34) -> (-79, 34) construction
  circle A6 centre (-63, 17) radius 4.5
  circle A7 centre (-51, 17) radius 4.5
  circle A8 centre (-63, 0) radius 4.5
  circle A9 centre (-51, 0) radius 4.5
  circle A10 centre (-63, -17) radius 4.5
  circle A11 centre (-51, -17) radius 4.5
  line L4 (-49.3079, 34.1971) -> (-49.3079, 18.6542) construction
  line L5 (-49.3079, 18.6542) -> (-53.9311, 18.6542) construction
  line L6 (-53.9311, 18.6542) -> (-53.9311, 34.1971) construction
  line L7 (-53.9311, 34.1971) -> (-49.3079, 34.1971) construction
  line L8 (-61.0894, 34.5417) -> (-61.0894, 18.9987) construction
  line L9 (-61.0894, 18.9987) -> (-65.7126, 18.9987) construction
  line L10 (-65.7126, 18.9987) -> (-65.7126, 34.5417) construction
  line L11 (-65.7126, 34.5417) -> (-61.0894, 34.5417) construction
  line L12 (-39.5338, 17.8903) -> (-39.5338, 15.2638) construction
  line L13 (-39.5338, 15.2638) -> (-43.0452, 15.2638) construction
  line L14 (-43.0452, 15.2638) -> (-43.0452, 17.8903) construction
  line L15 (-43.0452, 17.8903) -> (-39.5338, 17.8903) construction
  line L16 (-39.3872, 1.4286) -> (-39.3872, -1.1978) construction
  line L17 (-39.3872, -1.1978) -> (-42.8985, -1.1978) construction
  line L18 (-42.8985, -1.1978) -> (-42.8985, 1.4286) construction
  line L19 (-42.8985, 1.4286) -> (-39.3872, 1.4286) construction
  line L20 (-42.9654, -16.3361) -> (-39.454, -16.3361) construction
  line L21 (-39.454, -16.3361) -> (-39.454, -18.9625) construction
  line L22 (-39.454, -18.9625) -> (-42.9654, -18.9625) construction
  line L23 (-42.9654, -18.9625) -> (-42.9654, -16.3361) construction
  line L24 (-43.0452, 15.6524) -> (-43.0452, 17.3599)
  line L25 (-43.0452, 17.3599) -> (-42.6878, 17.3599)
  line L26 (-42.6878, 17.3599) -> (-42.6878, 16.7245)
  line L27 (-42.6878, 16.7245) -> (-40.3422, 16.7245)
  line L28 (-40.3422, 16.7245) -> (-40.3422, 17.3599)
  line L29 (-40.3422, 17.3599) -> (-40.0217, 17.3599)
  spline S0 degree 2 poles (-40.0217, 17.3599) (-40.0217, 16.9997) (-39.8175, 16.6593) (-39.5338, 16.6366) knots 0 0 0 1 2 2 2
  line L30 (-39.5338, 16.6366) -> (-39.5338, 16.2736)
  line L31 (-39.5338, 16.2736) -> (-42.6878, 16.2736)
  line L32 (-42.6878, 16.2736) -> (-42.6878, 15.6524)
  line L33 (-42.6878, 15.6524) -> (-43.0452, 15.6524)
  line L34 (-42.9609, -0.9851) -> (-42.9609, 1.1733)
  line L35 (-42.9609, 1.1733) -> (-42.4646, 1.1733)
  spline S1 degree 2 poles (-42.4646, 1.1733) (-42.2462, 0.9407) (-41.8406, 0.5266) (-41.6222, 0.3281) knots 0 0 0 1 2 2 2
  spline S2 degree 2 poles (-41.6222, 0.3281) (-41.1826, -0.0718) (-40.655, -0.364) (-40.3742, -0.364) knots 0 0 0 1 2 2 2
  spline S3 degree 2 poles (-40.3742, -0.364) (-40.2268, -0.364) (-40.0055, -0.2732) (-39.9346, -0.1909) knots 0 0 0 1 2 2 2
  spline S4 degree 2 poles (-39.9346, -0.1909) (-39.8637, -0.1087) (-39.7928, 0.1069) (-39.7928, 0.2373) knots 0 0 0 1 2 2 2
  spline S5 degree 2 poles (-39.7928, 0.2373) (-39.7928, 0.3621) (-39.8552, 0.6174) (-39.9034, 0.7337) knots 0 0 0 1 2 2 2
  spline S6 degree 2 poles (-39.9034, 0.7337) (-39.9431, 0.833) (-40.0566, 1.0173) (-40.0963, 1.074) knots 0 0 0 1 2 2 2
  line L36 (-40.0963, 1.074) -> (-40.0963, 1.0996)
  line L37 (-40.0963, 1.0996) -> (-39.5971, 1.0996)
  spline S7 degree 2 poles (-39.5971, 1.0996) (-39.5262, 0.9549) (-39.3872, 0.4359) (-39.3872, 0.2033) knots 0 0 0 1 2 2 2
  spline S8 degree 2 poles (-39.3872, 0.2033) (-39.3872, -0.2874) (-39.9062, -0.8405) (-40.3487, -0.8405) knots 0 0 0 1 2 2 2
  spline S9 degree 2 poles (-40.3487, -0.8405) (-40.5558, -0.8405) (-40.9018, -0.744) (-41.0493, -0.6589) knots 0 0 0 1 2 2 2
  spline S10 degree 2 poles (-41.0493, -0.6589) (-41.2024, -0.5738) (-41.5031, -0.3271) (-41.6477, -0.1909) knots 0 0 0 1 2 2 2
  spline S11 degree 2 poles (-41.6477, -0.1909) (-41.8888, 0.0303) (-42.405, 0.572) (-42.5554, 0.7337) knots 0 0 0 1 2 2 2
  line L38 (-42.5554, 0.7337) -> (-42.5554, -0.9851)
  line L39 (-42.5554, -0.9851) -> (-42.9609, -0.9851)
  spline S12 degree 2 poles (-39.8596, -17.5358) (-39.8596, -17.4082) (-39.922, -17.1557) (-39.9703, -17.0338) knots 0 0 0 1 2 2 2
  spline S13 degree 2 poles (-39.9703, -17.0338) (-40.0185, -16.9203) (-40.1206, -16.753) (-40.166, -16.6878) knots 0 0 0 1 2 2 2
  line L40 (-40.166, -16.6878) -> (-40.166, -16.6594)
  line L41 (-40.166, -16.6594) -> (-39.6696, -16.6594)
  spline S14 degree 2 poles (-39.6696, -16.6594) (-39.5874, -16.8126) (-39.454, -17.3373) (-39.454, -17.5727) knots 0 0 0 1 2 2 2
  spline S15 degree 2 poles (-39.454, -17.5727) (-39.454, -17.8109) (-39.5505, -18.1655) (-39.6526, -18.3101) knots 0 0 0 1 2 2 2
  spline S16 degree 2 poles (-39.6526, -18.3101) (-39.7632, -18.4633) (-40.0837, -18.6221) (-40.2993, -18.6221) knots 0 0 0 1 2 2 2
  spline S17 degree 2 poles (-40.2993, -18.6221) (-40.5886, -18.6221) (-41.0254, -18.242) (-41.0821, -17.9754) knots 0 0 0 1 2 2 2
  line L42 (-41.0821, -17.9754) -> (-41.1161, -17.9754)
  spline S18 degree 2 poles (-41.1161, -17.9754) (-41.1388, -18.0861) (-41.2409, -18.3385) (-41.343, -18.4463) knots 0 0 0 1 2 2 2
  spline S19 degree 2 poles (-41.343, -18.4463) (-41.4423, -18.554) (-41.76, -18.6902) (-41.9897, -18.6902) knots 0 0 0 1 2 2 2
  spline S20 degree 2 poles (-41.9897, -18.6902) (-42.2251, -18.6902) (-42.625, -18.5285) (-42.7782, -18.381) knots 0 0 0 1 2 2 2
  spline S21 degree 2 poles (-42.7782, -18.381) (-42.937, -18.2279) (-43.1015, -17.7939) (-43.1015, -17.5188) knots 0 0 0 1 2 2 2
  spline S22 degree 2 poles (-43.1015, -17.5188) (-43.1015, -17.255) (-42.9739, -16.7388) (-42.886, -16.563) knots 0 0 0 1 2 2 2
  line L43 (-42.886, -16.563) -> (-42.3896, -16.563)
  line L44 (-42.3896, -16.563) -> (-42.3896, -16.597)
  spline S23 degree 2 poles (-42.3896, -16.597) (-42.4974, -16.7445) (-42.6959, -17.2437) (-42.6959, -17.4904) knots 0 0 0 1 2 2 2
  spline S24 degree 2 poles (-42.6959, -17.4904) (-42.6959, -17.6351) (-42.6052, -17.9244) (-42.5002, -18.0208) knots 0 0 0 1 2 2 2
  spline S25 degree 2 poles (-42.5002, -18.0208) (-42.3953, -18.1144) (-42.1457, -18.2137) (-41.9557, -18.2137) knots 0 0 0 1 2 2 2
  spline S26 degree 2 poles (-41.9557, -18.2137) (-41.7656, -18.2137) (-41.5189, -18.1031) (-41.448, -18.0038) knots 0 0 0 1 2 2 2
  spline S27 degree 2 poles (-41.448, -18.0038) (-41.3771, -17.9045) (-41.3232, -17.6351) (-41.3232, -17.4762) knots 0 0 0 1 2 2 2
  line L45 (-41.3232, -17.4762) -> (-41.3232, -17.2777)
  line L46 (-41.3232, -17.2777) -> (-40.9346, -17.2777)
  line L47 (-40.9346, -17.2777) -> (-40.9346, -17.4337)
  spline S28 degree 2 poles (-40.9346, -17.4337) (-40.9346, -17.7485) (-40.6339, -18.1456) (-40.3475, -18.1456) knots 0 0 0 1 2 2 2
  spline S29 degree 2 poles (-40.3475, -18.1456) (-40.2142, -18.1456) (-40.0241, -18.0435) (-39.9674, -17.9613) knots 0 0 0 1 2 2 2
  spline S30 degree 2 poles (-39.9674, -17.9613) (-39.9079, -17.8733) (-39.8596, -17.6578) (-39.8596, -17.5358) knots 0 0 0 1 2 2 2
  spline S31 degree 2 poles (-63.7879, 33.5763) (-63.7879, 33.8521) (-63.6727, 34.2391) (-63.5903, 34.4099) knots 0 0 0 1 2 2 2
  line L48 (-63.5903, 34.4099) -> (-63.1663, 34.4099)
  line L49 (-63.1663, 34.4099) -> (-63.1663, 34.3852)
  spline S32 degree 2 poles (-63.1663, 34.3852) (-63.3227, 34.2185) (-63.4956, 33.7965) (-63.4956, 33.601) knots 0 0 0 1 2 2 2
  spline S33 degree 2 poles (-63.4956, 33.601) (-63.4956, 33.3211) (-63.2631, 33.035) (-63.0716, 33.035) knots 0 0 0 1 2 2 2
  spline S34 degree 2 poles (-63.0716, 33.035) (-62.9193, 33.035) (-62.7299, 33.1852) (-62.6826, 33.3478) knots 0 0 0 1 2 2 2
  spline S35 degree 2 poles (-62.6826, 33.3478) (-62.6497, 33.4652) (-62.6044, 33.6607) (-62.5673, 33.8068) knots 0 0 0 1 2 2 2
  spline S36 degree 2 poles (-62.5673, 33.8068) (-62.5323, 33.9386) (-62.4274, 34.1465) (-62.343, 34.2267) knots 0 0 0 1 2 2 2
  spline S37 degree 2 poles (-62.343, 34.2267) (-62.2586, 34.305) (-62.0322, 34.3914) (-61.884, 34.3914) knots 0 0 0 1 2 2 2
  spline S38 degree 2 poles (-61.884, 34.3914) (-61.5752, 34.3914) (-61.1574, 33.9098) (-61.1574, 33.5372) knots 0 0 0 1 2 2 2
  spline S39 degree 2 poles (-61.1574, 33.5372) (-61.1574, 33.3231) (-61.2418, 32.9444) (-61.322, 32.7818) knots 0 0 0 1 2 2 2
  line L50 (-61.322, 32.7818) -> (-61.7255, 32.7818)
  line L51 (-61.7255, 32.7818) -> (-61.7255, 32.8065)
  spline S40 degree 2 poles (-61.7255, 32.8065) (-61.6143, 32.9279) (-61.4497, 33.3067) (-61.4497, 33.5146) knots 0 0 0 1 2 2 2
  spline S41 degree 2 poles (-61.4497, 33.5146) (-61.4497, 33.7492) (-61.6699, 34.0394) (-61.849, 34.0394) knots 0 0 0 1 2 2 2
  spline S42 degree 2 poles (-61.849, 34.0394) (-62.0095, 34.0394) (-62.2009, 33.8686) (-62.2442, 33.708) knots 0 0 0 1 2 2 2
  spline S43 degree 2 poles (-62.2442, 33.708) (-62.273, 33.601) (-62.3471, 33.2902) (-62.378, 33.1873) knots 0 0 0 1 2 2 2
  spline S44 degree 2 poles (-62.378, 33.1873) (-62.4582, 32.9259) (-62.7814, 32.683) (-63.0181, 32.683) knots 0 0 0 1 2 2 2
  spline S45 degree 2 poles (-63.0181, 32.683) (-63.1684, 32.683) (-63.4565, 32.8044) (-63.5574, 32.9135) knots 0 0 0 1 2 2 2
  spline S46 degree 2 poles (-63.5574, 32.9135) (-63.6685, 33.035) (-63.7879, 33.3437) (-63.7879, 33.5763) knots 0 0 0 1 2 2 2
  spline S47 degree 2 poles (-63.5409, 31.3018) (-63.5697, 31.3409) (-63.6727, 31.4727) (-63.7035, 31.5344) knots 0 0 0 1 2 2 2
  spline S48 degree 2 poles (-63.7035, 31.5344) (-63.7488, 31.6188) (-63.7962, 31.7773) (-63.7962, 31.9214) knots 0 0 0 1 2 2 2
  spline S49 degree 2 poles (-63.7962, 31.9214) (-63.7962, 32.0387) (-63.7077, 32.2507) (-63.6274, 32.331) knots 0 0 0 1 2 2 2
  spline S50 degree 2 poles (-63.6274, 32.331) (-63.5492, 32.4072) (-63.3186, 32.4998) (-63.191, 32.4998) knots 0 0 0 1 2 2 2
  spline S51 degree 2 poles (-63.191, 32.4998) (-62.9934, 32.4998) (-62.7135, 32.3331) (-62.6332, 32.1519) knots 0 0 0 1 2 2 2
  spline S52 degree 2 poles (-62.6332, 32.1519) (-62.5591, 31.9914) (-62.5035, 31.555) (-62.4891, 31.3018) knots 0 0 0 1 2 2 2
  line L52 (-62.4891, 31.3018) -> (-62.4274, 31.3018)
  spline S53 degree 2 poles (-62.4274, 31.3018) (-62.3162, 31.3018) (-62.1783, 31.3698) (-62.1392, 31.4315) knots 0 0 0 1 2 2 2
  spline S54 degree 2 poles (-62.1392, 31.4315) (-62.1001, 31.4933) (-62.0754, 31.6703) (-62.0754, 31.765) knots 0 0 0 1 2 2 2
  spline S55 degree 2 poles (-62.0754, 31.765) (-62.0754, 31.8761) (-62.1413, 32.1766) (-62.2051, 32.3269) knots 0 0 0 1 2 2 2
  line L53 (-62.2051, 32.3269) -> (-62.2051, 32.3454)
  line L54 (-62.2051, 32.3454) -> (-61.8778, 32.3454)
  spline S56 degree 2 poles (-61.8778, 32.3454) (-61.8531, 32.2569) (-61.7913, 31.9255) (-61.7913, 31.7629) knots 0 0 0 1 2 2 2
  spline S57 degree 2 poles (-61.7913, 31.7629) (-61.7913, 31.5653) (-61.8531, 31.2957) (-61.9334, 31.1886) knots 0 0 0 1 2 2 2
  spline S58 degree 2 poles (-61.9334, 31.1886) (-62.0116, 31.0836) (-62.2606, 30.9807) (-62.4397, 30.9807) knots 0 0 0 1 2 2 2
  line L55 (-62.4397, 30.9807) -> (-63.7426, 30.9807)
  line L56 (-63.7426, 30.9807) -> (-63.7426, 31.3018)
  line L57 (-63.7426, 31.3018) -> (-63.5409, 31.3018)
  line L58 (-63.2733, 31.3018) -> (-62.7444, 31.3018)
  spline S59 degree 2 poles (-62.7444, 31.3018) (-62.7546, 31.4171) (-62.7896, 31.765) (-62.8226, 31.8741) knots 0 0 0 1 2 2 2
  spline S60 degree 2 poles (-62.8226, 31.8741) (-62.8617, 32.0017) (-63.0243, 32.1684) (-63.1684, 32.1684) knots 0 0 0 1 2 2 2
  spline S61 degree 2 poles (-63.1684, 32.1684) (-63.333, 32.1684) (-63.4998, 31.9831) (-63.4998, 31.8061) knots 0 0 0 1 2 2 2
  spline S62 degree 2 poles (-63.4998, 31.8061) (-63.4998, 31.6559) (-63.3701, 31.4089) (-63.2733, 31.3018) knots 0 0 0 1 2 2 2
  line L59 (-63.7426, 28.3687) -> (-62.6394, 28.3687)
  spline S63 degree 2 poles (-62.6394, 28.3687) (-62.5076, 28.3687) (-62.2833, 28.3893) (-62.2215, 28.4222) knots 0 0 0 1 2 2 2
  spline S64 degree 2 poles (-62.2215, 28.4222) (-62.1536, 28.4551) (-62.0877, 28.5807) (-62.0877, 28.6898) knots 0 0 0 1 2 2 2
  spline S65 degree 2 poles (-62.0877, 28.6898) (-62.0877, 28.7886) (-62.2092, 29.015) (-62.3244, 29.1344) knots 0 0 0 1 2 2 2
  spline S66 degree 2 poles (-62.3244, 29.1344) (-62.3533, 29.1323) (-62.4335, 29.1282) (-62.4871, 29.1282) knots 0 0 0 1 2 2 2
  line L60 (-62.4871, 29.1282) -> (-63.7426, 29.1282)
  line L61 (-63.7426, 29.1282) -> (-63.7426, 29.4493)
  line L62 (-63.7426, 29.4493) -> (-62.6394, 29.4493)
  spline S67 degree 2 poles (-62.6394, 29.4493) (-62.5076, 29.4493) (-62.2833, 29.4699) (-62.2215, 29.5028) knots 0 0 0 1 2 2 2
  spline S68 degree 2 poles (-62.2215, 29.5028) (-62.1536, 29.5358) (-62.0877, 29.6613) (-62.0877, 29.7704) knots 0 0 0 1 2 2 2
  spline S69 degree 2 poles (-62.0877, 29.7704) (-62.0877, 29.8733) (-62.2174, 30.1018) (-62.3183, 30.2088) knots 0 0 0 1 2 2 2
  line L63 (-62.3183, 30.2088) -> (-63.7426, 30.2088)
  line L64 (-63.7426, 30.2088) -> (-63.7426, 30.53)
  line L65 (-63.7426, 30.53) -> (-61.8366, 30.53)
  line L66 (-61.8366, 30.53) -> (-61.8366, 30.2088)
  line L67 (-61.8366, 30.2088) -> (-62.0466, 30.2088)
  spline S70 degree 2 poles (-62.0466, 30.2088) (-61.921, 30.0833) (-61.7831, 29.8363) (-61.7831, 29.6881) knots 0 0 0 1 2 2 2
  spline S71 degree 2 poles (-61.7831, 29.6881) (-61.7831, 29.5193) (-61.9375, 29.2579) (-62.1124, 29.19) knots 0 0 0 1 2 2 2
  spline S72 degree 2 poles (-62.1124, 29.19) (-61.9498, 29.0438) (-61.7831, 28.768) (-61.7831, 28.6075) knots 0 0 0 1 2 2 2
  spline S73 degree 2 poles (-61.7831, 28.6075) (-61.7831, 28.484) (-61.8593, 28.2822) (-61.9457, 28.2081) knots 0 0 0 1 2 2 2
  spline S74 degree 2 poles (-61.9457, 28.2081) (-62.0322, 28.132) (-62.2915, 28.0476) (-62.4871, 28.0476) knots 0 0 0 1 2 2 2
  line L68 (-62.4871, 28.0476) -> (-63.7426, 28.0476)
  line L69 (-63.7426, 28.0476) -> (-63.7426, 28.3687)
  spline S75 degree 2 poles (-62.7382, 25.9995) (-63.2157, 25.9995) (-63.7797, 26.4544) (-63.7797, 26.8023) knots 0 0 0 1 2 2 2
  spline S76 degree 2 poles (-63.7797, 26.8023) (-63.7797, 26.9443) (-63.7138, 27.1625) (-63.6459, 27.2757) knots 0 0 0 1 2 2 2
  line L70 (-63.6459, 27.2757) -> (-64.4445, 27.2757)
  line L71 (-64.4445, 27.2757) -> (-64.4445, 27.5968)
  line L72 (-64.4445, 27.5968) -> (-61.8366, 27.5968)
  line L73 (-61.8366, 27.5968) -> (-61.8366, 27.2757)
  line L74 (-61.8366, 27.2757) -> (-62.0363, 27.2757)
  spline S77 degree 2 poles (-62.0363, 27.2757) (-61.9272, 27.1563) (-61.7831, 26.864) (-61.7831, 26.6932) knots 0 0 0 1 2 2 2
  spline S78 degree 2 poles (-61.7831, 26.6932) (-61.7831, 26.3659) (-62.3018, 25.9995) (-62.7382, 25.9995) knots 0 0 0 1 2 2 2
  spline S79 degree 2 poles (-62.7752, 26.3309) (-62.4479, 26.3309) (-62.0877, 26.5388) (-62.0877, 26.7714) knots 0 0 0 1 2 2 2
  spline S80 degree 2 poles (-62.0877, 26.7714) (-62.0877, 26.9073) (-62.2092, 27.1625) (-62.3039, 27.2757) knots 0 0 0 1 2 2 2
  line L75 (-62.3039, 27.2757) -> (-63.3866, 27.2757)
  spline S81 degree 2 poles (-63.3866, 27.2757) (-63.4462, 27.1501) (-63.4915, 26.9711) (-63.4915, 26.8558) knots 0 0 0 1 2 2 2
  spline S82 degree 2 poles (-63.4915, 26.8558) (-63.4915, 26.6067) (-63.1251, 26.3309) (-62.7752, 26.3309) knots 0 0 0 1 2 2 2
  line L76 (-63.7426, 25.3388) -> (-63.7426, 25.6599)
  line L77 (-63.7426, 25.6599) -> (-61.0894, 25.6599)
  line L78 (-61.0894, 25.6599) -> (-61.0894, 25.3388)
  line L79 (-61.0894, 25.3388) -> (-63.7426, 25.3388)
  spline S83 degree 2 poles (-63.7859, 24.04) (-63.7859, 24.4969) (-63.2733, 24.9992) (-62.7999, 24.9992) knots 0 0 0 1 2 2 2
  spline S84 degree 2 poles (-62.7999, 24.9992) (-62.3347, 24.9992) (-61.7831, 24.5113) (-61.7831, 24.1182) knots 0 0 0 1 2 2 2
  spline S85 degree 2 poles (-61.7831, 24.1182) (-61.7831, 23.9412) (-61.886, 23.6674) (-61.9951, 23.5666) knots 0 0 0 1 2 2 2
  spline S86 degree 2 poles (-61.9951, 23.5666) (-62.1042, 23.4636) (-62.4191, 23.3546) (-62.6476, 23.3546) knots 0 0 0 1 2 2 2
  line L80 (-62.6476, 23.3546) -> (-62.8226, 23.3546)
  line L81 (-62.8226, 23.3546) -> (-62.8226, 24.674)
  spline S87 degree 2 poles (-62.8226, 24.674) (-63.154, 24.674) (-63.5059, 24.3405) (-63.5059, 24.0441) knots 0 0 0 1 2 2 2
  spline S88 degree 2 poles (-63.5059, 24.0441) (-63.5059, 23.9391) (-63.4586, 23.7353) (-63.4215, 23.653) knots 0 0 0 1 2 2 2
  spline S89 degree 2 poles (-63.4215, 23.653) (-63.3804, 23.5666) (-63.3083, 23.4472) (-63.2754, 23.4081) knots 0 0 0 1 2 2 2
  line L82 (-63.2754, 23.4081) -> (-63.2754, 23.3895)
  line L83 (-63.2754, 23.3895) -> (-63.6253, 23.3895)
  spline S90 degree 2 poles (-63.6253, 23.3895) (-63.648, 23.4451) (-63.7138, 23.6139) (-63.7324, 23.6798) knots 0 0 0 1 2 2 2
  spline S91 degree 2 poles (-63.7324, 23.6798) (-63.7591, 23.7724) (-63.7859, 23.9247) (-63.7859, 24.04) knots 0 0 0 1 2 2 2
  spline S92 degree 2 poles (-62.5776, 23.6674) (-62.4479, 23.6715) (-62.2586, 23.7251) (-62.1948, 23.7765) knots 0 0 0 1 2 2 2
  spline S93 degree 2 poles (-62.1948, 23.7765) (-62.1227, 23.8321) (-62.0466, 24.007) (-62.0466, 24.1367) knots 0 0 0 1 2 2 2
  spline S94 degree 2 poles (-62.0466, 24.1367) (-62.0466, 24.2643) (-62.1227, 24.4434) (-62.1968, 24.5175) knots 0 0 0 1 2 2 2
  spline S95 degree 2 poles (-62.1968, 24.5175) (-62.273, 24.5896) (-62.4562, 24.6637) (-62.5776, 24.674) knots 0 0 0 1 2 2 2
  line L84 (-62.5776, 24.674) -> (-62.5776, 23.6674)
  spline S96 degree 2 poles (-51.181, 32.217) (-51.3704, 32.217) (-51.6606, 32.3611) (-51.7553, 32.4805) knots 0 0 0 1 2 2 2
  spline S97 degree 2 poles (-51.7553, 32.4805) (-51.8664, 32.6246) (-51.9611, 32.9518) (-51.9611, 33.2112) knots 0 0 0 1 2 2 2
  line L85 (-51.9611, 33.2112) -> (-51.9611, 33.9398)
  line L86 (-51.9611, 33.9398) -> (-49.4211, 33.9398)
  line L87 (-49.4211, 33.9398) -> (-49.4211, 33.2668)
  spline S98 degree 2 poles (-49.4211, 33.2668) (-49.4211, 32.9951) (-49.4561, 32.7234) (-49.524, 32.5999) knots 0 0 0 1 2 2 2
  spline S99 degree 2 poles (-49.524, 32.5999) (-49.5961, 32.4619) (-49.8328, 32.3364) (-49.9933, 32.3364) knots 0 0 0 1 2 2 2
  spline S100 degree 2 poles (-49.9933, 32.3364) (-50.1724, 32.3364) (-50.4565, 32.5258) (-50.5367, 32.6925) knots 0 0 0 1 2 2 2
  line L88 (-50.5367, 32.6925) -> (-50.5491, 32.6925)
  spline S101 degree 2 poles (-50.5491, 32.6925) (-50.6108, 32.4661) (-50.9381, 32.217) (-51.181, 32.217) knots 0 0 0 1 2 2 2
  spline S102 degree 2 poles (-51.1954, 32.569) (-51.0513, 32.569) (-50.8661, 32.6513) (-50.8002, 32.7748) knots 0 0 0 1 2 2 2
  spline S103 degree 2 poles (-50.8002, 32.7748) (-50.7591, 32.8551) (-50.7344, 33.0445) (-50.7344, 33.2194) knots 0 0 0 1 2 2 2
  line L89 (-50.7344, 33.2194) -> (-50.7344, 33.6023)
  line L90 (-50.7344, 33.6023) -> (-51.673, 33.6023)
  line L91 (-51.673, 33.6023) -> (-51.673, 33.3285)
  spline S104 degree 2 poles (-51.673, 33.3285) (-51.673, 33.1062) (-51.6318, 32.851) (-51.5659, 32.7522) knots 0 0 0 1 2 2 2
  spline S105 degree 2 poles (-51.5659, 32.7522) (-51.498, 32.6575) (-51.3292, 32.569) (-51.1954, 32.569) knots 0 0 0 1 2 2 2
  spline S106 degree 2 poles (-50.0407, 32.6884) (-49.9501, 32.6884) (-49.8143, 32.7501) (-49.7752, 32.818) knots 0 0 0 1 2 2 2
  spline S107 degree 2 poles (-49.7752, 32.818) (-49.7299, 32.9004) (-49.7093, 33.1) (-49.7093, 33.2791) knots 0 0 0 1 2 2 2
  line L92 (-49.7093, 33.2791) -> (-49.7093, 33.6023)
  line L93 (-49.7093, 33.6023) -> (-50.4524, 33.6023)
  line L94 (-50.4524, 33.6023) -> (-50.4524, 33.2194)
  spline S108 degree 2 poles (-50.4524, 33.2194) (-50.4524, 33.0609) (-50.4194, 32.9107) (-50.368, 32.8304) knots 0 0 0 1 2 2 2
  spline S109 degree 2 poles (-50.368, 32.8304) (-50.3186, 32.7522) (-50.1601, 32.6884) (-50.0407, 32.6884) knots 0 0 0 1 2 2 2
  line L95 (-51.9611, 31.5789) -> (-51.9611, 31.9)